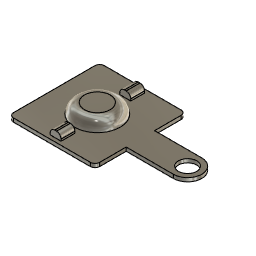
Positive Connector (Autodesk Fusion 360 design; units mm, degrees)
Autodesk Fusion 360 part; units mm, degrees
sketch "Base" plane through (0, 0, 0) normal (0, 0, 1) x (1, 0, 0) in component "Positive Connector"
  line L0 (4.7, -4.95) -> (-4.7, -4.95)
  line L1 (-4.7, -4.95) -> (-4.7, 4.95)
  line L2 (-4.7, 4.95) -> (4.7, 4.95)
  line L3 (4.7, 4.95) -> (4.7, -4.95)
  line L4 (4.7, -4.95) -> (-4.7, 4.95) construction
  line L5 (-4.7, -4.95) -> (4.7, 4.95) construction
  dimension "d1" = 9.4
  dimension "d2" = 9.9
  constraint horizontal L0
  constraint perpendicular L0 L1
  constraint parallel L0 L2
  constraint parallel L1 L3
  constraint coincident L4 origin
  constraint coincident L5 origin
  measures "d1" distance of L1.end L2.end
  measures "d2" distance of L0.end L1.end
extrude "Extrude1" add sketch "Base" along normal blind 0.4 in component "Positive Connector"
fillet "Fillet1" radius 0.5 4 edges at (4.7, -4.95, 0.2) (4.7, 4.95, 0.2) (-4.7, 4.95, 0.2) (-4.7, -4.95, 0.2) in component "Positive Connector"
sketch "Connector" plane through (4.7, 0, 0) normal (1, 0, 0) x (0, 1, 0) in component "Positive Connector"
  line L0 (4.45, 0) -> (4.45, 0.4)
  line L1 (4.45, 0.4) -> (-4.45, 0.4)
  line L2 (-4.45, 0.4) -> (-4.45, 0)
  line L3 (-4.45, 0) -> (4.45, 0)
  line L4 (-4.45, 0.2) -> (4.45, 0.2) construction
  line L5 (1.55, 0) -> (-1.55, 0)
  line L6 (-1.55, 0) -> (-1.55, 0.4)
  line L7 (-1.55, 0.4) -> (1.55, 0.4)
  line L8 (1.55, 0.4) -> (1.55, 0)
  line L9 (1.55, 0) -> (-1.55, 0.4) construction
  line L10 (-1.55, 0) -> (1.55, 0.4) construction
  point P0 (0, 0.2)
  dimension "d6" = 3.1
  constraint midpoint L2 L4.start
  constraint midpoint L0 L4.end
  constraint horizontal L5
  constraint perpendicular L5 L6
  constraint parallel L5 L7
  constraint parallel L6 L8
  constraint coincident L9 P0
  constraint coincident L10 P0
  constraint midpoint L4 P0
  measures "d6" distance of L6.end L7.end
extrude "Extrude2" add sketch "Connector" along normal blind 6.7 contours L1 L3 L5 L6 L7 L8 in component "Positive Connector"
fillet "Fillet2" radius 1.55 2 edges at (11.4, -1.55, 0.2) (11.4, 1.55, 0.2) in component "Positive Connector"
sketch "Taps" plane through (0, 0, 0.4) normal (0, 0, 1) x (-1, 0, 0) in component "Positive Connector"
  arc A0 (-9.85, 1.55) -> (-9.85, -1.55) centre (-9.85, 0) ccw
  line L0 (-9.85, -1.55) -> (-4.7, -1.55)
  line L1 (-4.7, -1.55) -> (-4.7, -4.45)
  arc A1 (-4.7, -4.45) -> (-4.2, -4.95) centre (-4.2, -4.45) ccw
  line L2 (-4.2, -4.95) -> (4.2, -4.95)
  arc A2 (4.2, -4.95) -> (4.7, -4.45) centre (4.2, -4.45) ccw
  line L3 (4.7, -4.45) -> (4.7, 4.45)
  arc A3 (4.7, 4.45) -> (4.2, 4.95) centre (4.2, 4.45) ccw
  line L4 (4.2, 4.95) -> (-4.2, 4.95)
  arc A4 (-4.2, 4.95) -> (-4.7, 4.45) centre (-4.2, 4.45) ccw
  line L5 (-4.7, 4.45) -> (-4.7, 1.55)
  line L6 (-4.7, 1.55) -> (-9.85, 1.55)
  line L7 (4.7, 0) -> (-11.4, 0) construction
  line L8 (-9.85, -1.55) -> (-9.85, 1.55) construction
  circle A5 centre (-9.85, 0) radius 1
  line L9 (0, -4.95) -> (0, 4.95) construction
  circle A6 centre (0, 0) radius 2.5
  line L10 (-0.6, -3.05) -> (0.6, -3.05)
  line L11 (0.6, -3.05) -> (0.6, -4.55)
  line L12 (0.6, -4.55) -> (-0.6, -4.55)
  line L13 (-0.6, -4.55) -> (-0.6, -3.05)
  line L14 (-0.6, -3.05) -> (0.6, -4.55) construction
  line L15 (0.6, -3.05) -> (-0.6, -4.55) construction
  line L16 (-0.6, 4.55) -> (0.6, 4.55)
  line L17 (0.6, 4.55) -> (0.6, 3.05)
  line L18 (0.6, 3.05) -> (-0.6, 3.05)
  line L19 (-0.6, 3.05) -> (-0.6, 4.55)
  line L20 (-0.6, 4.55) -> (0.6, 3.05) construction
  line L21 (0.6, 4.55) -> (-0.6, 3.05) construction
  point P0 (0, -3.8)
  point P1 (0, 3.8)
  dimension "d10" = 1.55
  dimension "d11" = 2
  dimension "d12" = 5
  dimension "d13" = 1.2
  dimension "d14" = 1.5
  dimension "d15" = 0.4
  dimension "d16" = 1.2
  dimension "d17" = 1.5
  dimension "d18" = 0.4
  constraint midpoint L3 L7.start
  constraint midpoint A0 L7.end
  constraint coincident L0 A0.end
  constraint coincident L6 A0.start
  constraint perpendicular L6 L8
  constraint midpoint L8 A0.centre
  constraint midpoint L2 L9.start
  constraint midpoint L4 L9.end
  constraint coincident A6.centre origin
  constraint horizontal L10
  constraint perpendicular L10 L11
  constraint parallel L10 L12
  constraint parallel L11 L13
  constraint coincident L14 P0
  constraint coincident L15 P0
  constraint coincident L9 P0
  constraint horizontal L16
  constraint perpendicular L16 L17
  constraint parallel L16 L18
  constraint parallel L17 L19
  constraint coincident L20 P1
  constraint coincident L21 P1
  constraint coincident L9 P1
  measures "d10" distance of L7.end L8
  measures "d11" diameter of A5
  measures "d12" diameter of A6
  measures "d13" distance of L11.end L12.end
  measures "d14" distance of L10.end L11.end
  measures "d15" distance of L2 L12
  measures "d16" distance of L17.end L18.end
  measures "d17" distance of L16.end L17.end
  measures "d18" distance of L4 L16
extrude "Extrude3" cut sketch "Taps" against normal up to surface (0.4 mm away) contours A5 in component "Positive Connector"
extrude "Extrude4" add sketch "Taps" along normal blind 0.7 contours L10 L11 L12 L13 | L16 L17 L18 L19 in component "Positive Connector"
fillet "Fillet3" radius 0.5 4 edges at (0.6, 3.8, 1.1) (0.6, -3.8, 1.1) (-0.6, -3.8, 1.1) (-0.6, 3.8, 1.1) in component "Positive Connector"
extrude "Extrude5" add sketch "Taps" along normal blind 1.1 contours A6 in component "Positive Connector"
fillet "Fillet4" radius 1.1 1 edges at (2.3308, 0.904, 1.5) in component "Positive Connector"
component "Positive Connector" placed x (1, 0, 0) y (0, 1, 0) z (0, 0, 1) at (0, 0, 0)
named bodies: "Positive Connector"
